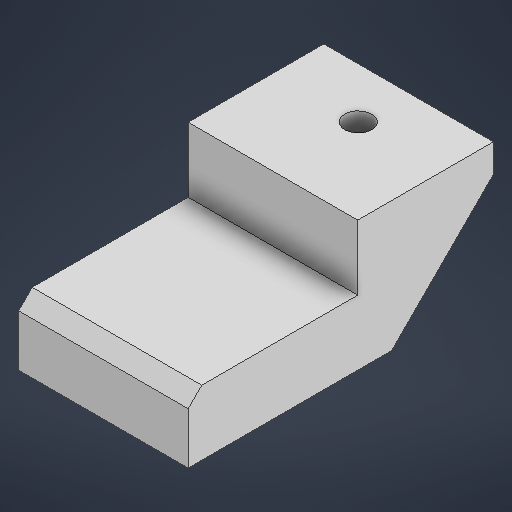
# Autodesk Inventor part: front wall bkt
Saved by Autodesk Inventor 2026.2 (Build 302298000, 298)
## iProperties
Created: 2026-01-18
Part Number: front wall bkt
Material: Generic
Document SubType Name: Modeling
Designer: User
Density: 1 g/cm^3
Appearance: Default
Author: User
Autodesk Inventor part; units mm, degrees
ref_plane "YZ Plane" through (0, 0, 0) normal (1, 0, 0) x (0, 1, 0)
ref_plane "XZ Plane" through (0, 0, 0) normal (0, 1, 0) x (-1, 0, 0)
sketch "Sketch1" plane through (0, 0, 0) normal (1, 0, 0) x (0, 1, 0)
  line L0 (0, 0) -> (9.5813, 0)
  line L1 (9.5813, 0) -> (9.5812, 23)
  line L2 (7.5812, 25) -> (0, 25)
  line L3 (0, 25) -> (0, 0)
  line L4 (9.5812, 23) -> (7.5812, 25)
  line L5 (0, 0) -> (19.1625, 0)
  line L6 (19.1625, 0) -> (19.1625, -20)
  line L7 (19.1625, -20) -> (15, -20)
  line L8 (0, -5) -> (0, 0)
  line L9 (19.1625, -20) -> (11.1625, -20)
  line L10 (15, -20) -> (0, -5)
  point P0 (9.5812, 25)
  point P1 (0, -20)
  dimension "d0" = 9.5813
  dimension "d1" = 25
  dimension "d2" = 2
  dimension "d3" = 2
  dimension "d4" = 20
  dimension "d5" = 19.1625
  dimension "d8" = 15
  dimension "d9" = 15
  constraints: 22 end point, 4 parallel, 4 point on line, 3 horizontal, 2 perpendicular
  measures "d0" distance of L2.end point (9.581, 25)
  measures "d1" distance of L2.end L0.start
  measures "d2" distance of L1.end point (9.581, 25)
  measures "d3" distance of L2.start point (9.581, 25)
  measures "d4" distance of L5.end L6.end
  measures "d5" distance of L6.end point (0, -20)
  measures "d8" distance of L7.end point (0, -20)
  measures "d9" distance of L8.start point (0, -20)
extrude "Extrusion1" add sketch "Sketch1" along normal blind 25
ref_plane "Work Plane1" through (0, 13.1625, 0) normal (0, 1, 0) x (1, 0, 0)
sketch "Sketch2" plane through (0, 13.1625, 0) normal (0, 1, 0) x (1, 0, 0)
  line L0 (20, 30.2149) -> (5, 30.2149)
  line L1 (5, 30.2149) -> (5, 7)
  line L2 (5, 7) -> (20, 7)
  line L3 (20, 7) -> (20, 30.2149)
  line L4 (25, 5) -> (25, 20) projected
  line L5 (0, 5) -> (0, 20) projected
  line L6 (0, 0) -> (25, 0) projected
  dimension "d13" = 5
  dimension "d14" = 5
  dimension "d15" = 7
  constraints: 8 end point, 2 parallel, 1 horizontal, 1 perpendicular
  measures "d13" distance between parallel lines of L4 L3
  measures "d14" distance between parallel lines of L5 L1
  measures "d15" distance between parallel lines of L6 L2
extrude "Extrusion2" cut sketch "Sketch2" against normal blind 25
sketch "Sketch3" plane through (0, 13.1625, 0) normal (0, -1, 0) x (1, 0, 0)
  circle A0 centre (12.5, -12.5813) radius 2
  line L0 (20, -7) -> (20, -18.1625) projected
  point P0 (0, 0)
  point P1 (20, -12.5813)
  dimension "d18" = 4
  dimension "d19" = 0
  constraints: 1 centre point, 1 midpoint
  measures "d18" diameter of A0
  measures "d19" vertical distance of A0.centre point (20, -12.581)
extrude "Extrusion3" cut sketch "Sketch3" against normal blind 25
chamfer "Chamfer1" distance 2 angle 45 1 edges at (10.5, 13.1625, -12.5813)
equation "\"d3\" = d2"
equation "\"d5\" = 2 * d0"
equation "\"d9\" = d8"
body "Solid1"
